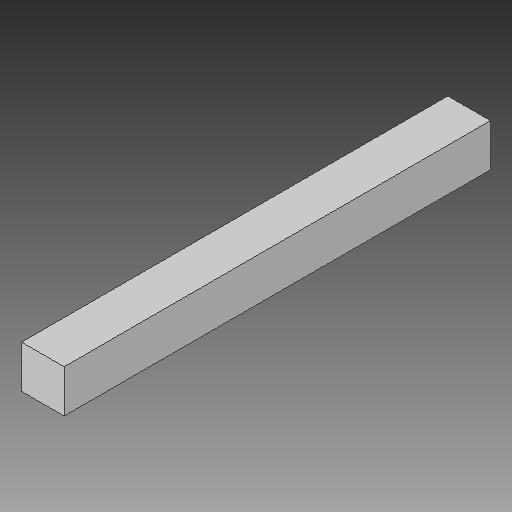
# Autodesk Inventor part: Кабельный канал 40х40х60
Saved by Autodesk Inventor 2019.3 (Build 233278000, 278)
## iProperties
Created: 2018-11-14
Part Number: Кабельный канал 40х40х60
Material: Типовые
Document SubType Name: Modeling
Designer: A.Vlaschuk
Density: 1 g/cm^3
Appearance: По умолчанию
Author: A.Vlaschuk
Autodesk Inventor part; units mm, degrees
ref_plane "YZ Plane" through (0, 0, 0) normal (1, 0, 0) x (0, 1, 0)
ref_plane "XZ Plane" through (0, 0, 0) normal (0, 1, 0) x (-1, 0, 0)
ref_plane "XY Plane" through (0, 0, 0) normal (0, 0, 1) x (1, 0, 0)
sketch "Эскиз1" plane through (0, 0, 0) normal (0, 0, 1) x (1, 0, 0)
  line L0 (0, 6.4238) -> (40, 6.4238)
  line L1 (40, 6.4238) -> (40, -33.5762)
  line L2 (40, -33.5762) -> (0, -33.5762)
  line L3 (0, -33.5762) -> (0, 6.4238)
  point P0 (0, 0)
  dimension "d0" = 40
  dimension "d1" = 40
  constraints: 8 end point, 2 parallel, 1 horizontal, 1 perpendicular
  measures "d0" distance of L1.end L2.end
  measures "d1" distance of L0.end L1.end
extrude "Выдавливание1" add sketch "Эскиз1" along normal blind 400
